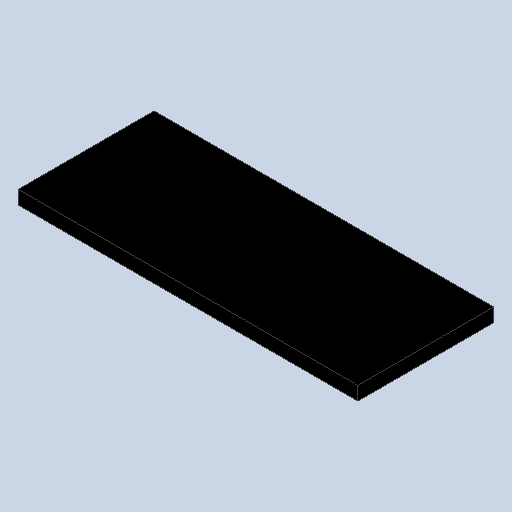
# Autodesk Inventor part: nickel strip
Saved by Autodesk Inventor 2025.2 (Build 292293000, 293)
## iProperties
Created: 2024-11-29
Part Number: nickel strip
Material: Generic
Document SubType Name: Modeling
Designer: cbast
Density: 1 g/cm^3
Appearance: Default
Author: cbast
Autodesk Inventor part; units mm, degrees
ref_plane "YZ Plane" through (0, 0, 0) normal (1, 0, 0) x (0, 1, 0)
ref_plane "XZ Plane" through (0, 0, 0) normal (0, 1, 0) x (-1, 0, 0)
ref_plane "XY Plane" through (0, 0, 0) normal (0, 0, 1) x (1, 0, 0)
sketch "Sketch1" plane through (0, 0, 0) normal (0, 1, 0) x (-1, 0, 0)
  line L0 (25.2468, 4.9196) -> (50.2468, 4.9196)
  line L1 (50.2468, 4.9196) -> (50.2468, -5.0804)
  line L2 (50.2468, -5.0804) -> (25.2468, -5.0804)
  line L3 (25.2468, -5.0804) -> (25.2468, 4.9196)
  line L4 (25.2468, 4.9196) -> (50.2468, -5.0804) construction
  line L5 (50.2468, 4.9196) -> (25.2468, -5.0804) construction
  point P0 (0, 0)
  point P1 (37.7468, -0.0804)
  dimension "d0" = 25
  dimension "d1" = 10
  constraints: 12 end point, 2 midpoint, 2 parallel, 1 horizontal, 1 perpendicular
  measures "d0" distance of L1.end L2.end
  measures "d1" distance of L0.end L1.end
extrude "Extrusion1" add sketch "Sketch1" along normal blind 1
body "Solid1"
